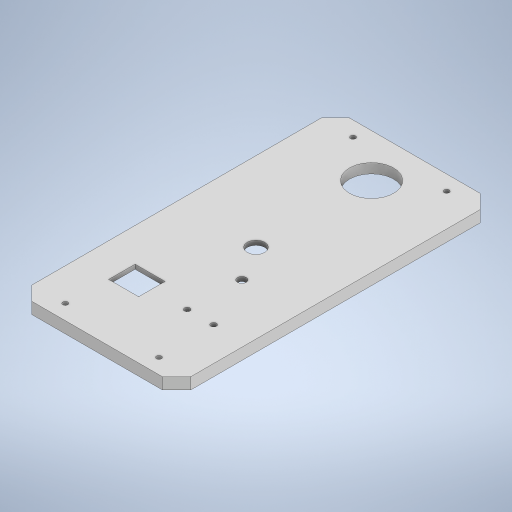
# Autodesk Inventor part: enclosed top
Saved by Autodesk Inventor 2023 (Build 270158000, 158)
## iProperties
Created: 2022-05-30
Part Number: enclosed top
Material: Generic
Document SubType Name: Modeling
Designer: Aakif
Density: 1 g/cm^3
Appearance: Default
Author: Aakif
Autodesk Inventor part; units mm, degrees
ref_plane "YZ Plane" through (0, 0, 0) normal (1, 0, 0) x (0, 1, 0)
ref_plane "XZ Plane" through (0, 0, 0) normal (0, 1, 0) x (-1, 0, 0)
ref_plane "XY Plane" through (0, 0, 0) normal (0, 0, 1) x (1, 0, 0)
sketch "Sketch1" plane through (0, 0, 0) normal (0, 1, 0) x (-1, 0, 0)
  line L0 (37, -90) -> (-37, -90)
  line L1 (-45, -82) -> (-45, 82)
  line L2 (-37, 90) -> (37, 90)
  line L3 (45, 82) -> (45, -82)
  line L4 (45, -90) -> (-45, 90) construction
  line L5 (-45, -90) -> (45, 90) construction
  line L6 (-37, -90) -> (-45, -82)
  line L7 (37, -90) -> (45, -82)
  line L8 (37, 90) -> (45, 82)
  line L9 (-45, 82) -> (-37, 90)
  line L10 (0, 0) -> (0, -65.5)
  circle A0 centre (0, -65.5) radius 12.5
  line L11 (0, 0) -> (0, 0)
  circle A1 centre (0, 0) radius 5
  line L12 (0, 0) -> (17.5, 0)
  line L13 (17.5, 0) -> (17.5, 50)
  line L14 (17.5, 50) -> (0, 50)
  line L15 (0, 50) -> (0, 0)
  line L16 (26, 42.5) -> (9, 42.5)
  line L17 (9, 42.5) -> (9, 57.5)
  line L18 (9, 57.5) -> (26, 57.5)
  line L19 (26, 57.5) -> (26, 42.5)
  line L20 (26, 42.5) -> (9, 57.5) construction
  line L21 (9, 42.5) -> (26, 57.5) construction
  line L22 (9, 50) -> (-11, 50)
  circle A2 centre (-11, 50) radius 1.6
  line L23 (-11, 50) -> (-26, 50)
  circle A3 centre (-26, 50) radius 1.6
  line L24 (41, -80.3431) -> (35.3431, -86)
  line L25 (35.3431, -86) -> (-35.3431, -86)
  line L26 (-35.3431, -86) -> (-41, -80.3431)
  line L27 (-41, -80.3431) -> (-41, 80.3431)
  line L28 (-41, 80.3431) -> (-35.3431, 86)
  line L29 (-35.3431, 86) -> (35.3431, 86)
  line L30 (35.3431, 86) -> (41, 80.3431)
  line L31 (41, 80.3431) -> (41, -80.3431)
  line L32 (45, -90) -> (35.8917, -82.1873)
  circle A4 centre (35.8917, -82.1873) radius 1.45
  circle A5 centre (35.8917, -82.1873) radius 4.45
  line L33 (22.0647, -90) -> (45, -90)
  line L34 (45, -90) -> (45, -77.0647)
  line L35 (45, -77.0647) -> (22.0647, -77.0647)
  line L36 (22.0647, -77.0647) -> (22.0647, -90)
  circle A6 centre (-35.8917, -82.1873) radius 1.45
  circle A7 centre (-35.8917, -82.1873) radius 4.45
  line L37 (-45, -77.0647) -> (-22.0647, -77.0647)
  line L38 (-22.0647, -77.0647) -> (-22.0647, -90)
  circle A8 centre (35.8917, 82.1873) radius 1.45
  circle A9 centre (35.8917, 82.1873) radius 4.45
  line L39 (45, 77.0647) -> (22.0647, 77.0647)
  line L40 (22.0647, 77.0647) -> (22.0647, 90)
  circle A10 centre (-35.8917, 82.1873) radius 4.45
  circle A11 centre (-35.8917, 82.1873) radius 1.45
  line L41 (-45, 77.0647) -> (-22.0647, 77.0647)
  line L42 (-22.0647, 77.0647) -> (-22.0647, 90)
  line L43 (-22.0647, -90) -> (-45, -90)
  line L44 (-45, -90) -> (-45, -77.0647)
  line L45 (-22.0647, 90) -> (-45, 90)
  line L46 (-45, 90) -> (-45, 77.0647)
  line L47 (22.0647, 90) -> (45, 90)
  line L48 (45, 90) -> (45, 77.0647)
  line L49 (0, 0) -> (0, 20)
  line L50 (0, 0) -> (20, 0) construction
  line L51 (0, 20) -> (-12, 20)
  circle A12 centre (-12, 20) radius 2.5
  line L52 (0, 86) -> (12.5, 86)
  line L53 (0, 86) -> (-12.5, 86)
  circle A13 centre (12.5, 86) radius 1.5
  circle A14 centre (-12.5, 86) radius 1.5
  line L54 (0, -65.5) -> (14, -65.5)
  line L55 (0, -65.5) -> (14, -65.5) construction
  line L56 (0, -65.5) -> (-14, -65.5)
  line L57 (0, -65.5) -> (14, -65.5) construction
  circle A15 centre (14, -65.5) radius 0.95
  circle A16 centre (-14, -65.5) radius 0.95
  circle A17 centre (0, -65.5) radius 15.45
  point P0 (22.0647, -86)
  point P1 (-22.0647, -86)
  point P2 (-22.0647, -81.5147)
  point P3 (-26.5147, -77.0647)
  point P4 (-41, -77.0647)
  point P5 (-41, 77.0647)
  point P6 (-26.5147, 77.0647)
  point P7 (-22.0647, 81.5147)
  point P8 (-22.0647, 86)
  point P9 (22.0647, 86)
  point P10 (22.0647, 81.5147)
  point P11 (26.5147, 77.0647)
  point P12 (41, 77.0647)
  point P13 (41, -77.0647)
  point P14 (26.5147, -77.0647)
  point P15 (22.0647, -81.5147)
  point P16 (5, 0)
  point P17 (0, 5)
  point P18 (9, 50)
  point P19 (17.5, 42.5)
  dimension "d0" = 90
  dimension "d1" = 180
  dimension "d2" = 8
  dimension "d3" = 8
  dimension "d4" = 8
  dimension "d5" = 8
  dimension "d6" = 8
  dimension "d7" = 8
  dimension "d8" = 8
  dimension "d9" = 8
  dimension "d10" = 65.5
  dimension "d11" = 25
  dimension "d12" = 0
  dimension "d13" = 10
  dimension "d14" = 17.5
  dimension "d15" = 50
  dimension "d16" = 17
  dimension "d17" = 15
  dimension "d20" = 20
  dimension "d21" = 3.2
  dimension "d22" = 15
  dimension "d23" = 3.2
  dimension "d24" = 4
  dimension "d25" = 12
  dimension "d26" = 2.9
  dimension "d27" = 3
  dimension "d57" = 20
  dimension "d58" = 90
  dimension "d59" = 12
  dimension "d60" = 90
  dimension "d61" = 5
  dimension "d70" = 12.5
  dimension "d71" = 12.5
  dimension "d72" = 3
  dimension "d73" = 3
  dimension "d74" = 14
  dimension "d75" = 0
  dimension "d76" = 14
  dimension "d77" = 180
  dimension "d78" = 1.9
  dimension "d79" = 1.9
  dimension "d80" = 30.9
  constraints: 116 end point, 18 centre point, 14 symmetric about line, 13 point on line, 11 coincident, 10 horizontal, 10 parallel, 8 perpendicular, 6 midpoint, 3 equal length, 2 collinear, 13 other
  measures "d0" distance of L4.end L5.end
  measures "d1" distance of L5.start L4.end
  measures "d2" distance of L0.end L5.start
  measures "d3" distance of L1.start L5.start
  measures "d4" distance of L0.start L4.start
  measures "d5" distance of L3.end L4.start
  measures "d6" distance of L2.end L5.end
  measures "d7" distance of L3.start L5.end
  measures "d8" distance of L1.end L4.end
  measures "d9" distance of L2.start L4.end
  measures "d10" distance of L10.start L10.end
  measures "d11" diameter of A0
  measures "d12" distance of L10.start L11.end
  measures "d13" diameter of A1
  measures "d14" distance of L14.end L13.end
  measures "d15" distance of L13.end L12.end
  measures "d16" distance of L17.end L18.end
  measures "d17" distance of L16.end L17.end
  measures "d20" distance of L22.start L22.end
  measures "d21" diameter of A2
  measures "d22" distance of L23.start L23.end
  measures "d23" diameter of A3
  measures "d24" distance between parallel lines of L7 L24
  measures "d25" distance of L4.start L32.end
  measures "d26" diameter of A4
  measures "d27" radial gap between concentric circles of A4 A5
  measures "d57" distance of L49.start L49.end
  measures "d58" angle of L50 L49
  measures "d59" distance of L49.end L51.end
  measures "d60" angle of L51 L49
  measures "d61" diameter of A12
  measures "d70" distance of L52.start L52.end
  measures "d71" distance of L52.start L53.end
  measures "d72" diameter of A13
  measures "d73" diameter of A14
  measures "d74" distance of L54.start L54.end
  measures "d75" distance between parallel lines of L54 L55
  measures "d76" distance of L54.start L56.end
  measures "d77" angle of L56 L57
  measures "d78" diameter of A15
  measures "d79" diameter of A16
  measures "d80" diameter of A17
extrude "Extrusion1" add sketch "Sketch1" along normal blind 2.5 contours L0 L36 L25 A5 L32 L7 | L0 L38 L25 L36 | L32 A5 L24 L31 L35 L3 L7 | L0 L6 L1 L37 L27 L26 A7 L25 L38 | L36 L35 L31 L24 A5 L25 | L25 L38 L37 L27 L41 L42 L29 A14 A13 L40 L39 L31 L35 L36 | A5 L25 L24 L32 | L32 L24 A5 | L25 A7 L26 L27 L37 L38 | A5 L24 L25 | L35 L31 L39 L3 | A7 L26 L25 | L25 L26 A7 | L39 L31 L30 A9 L29 L40 L2 L8 L3 | L1 L41 L27 L37 | L39 L40 L29 A9 L30 L31 | L1 L9 L2 L42 L29 A10 L28 L27 L41 | L27 L28 A10 L29 L42 L41 | A9 L29 L30 | L30 L29 A9 | L29 A13 A14 L42 L2 L40 | A10 L29 L28 | L28 L29 A10 | A13 L29 | L29 A13 | A14 L29 | L29 A14 | A1 L15 L14 L17 L16 L13 L12 | A4 | A6 | A8 | A11 | A12 | A15 | A16 | A17
sketch "Sketch2" plane through (0, 0, 0) normal (0, -1, 0) x (1, 0, 0)
  line L0 (-26, 57.5) -> (-26, 42.5) projected
  line L1 (-26, 50) -> (-5, 50)
  circle A0 centre (-5, 50) radius 1.45
  circle A1 centre (-5, 50) radius 3.45
  circle A2 centre (0, -65.5) radius 12.5 projected
  line L2 (0, -65.5) -> (-14, -65.5)
  line L3 (0, -65.5) -> (14, -65.5)
  circle A3 centre (-14, -65.5) radius 0.95
  circle A4 centre (14, -65.5) radius 0.95
  circle A5 centre (-14, -65.5) radius 1.45
  circle A6 centre (14, -65.5) radius 1.45
  line L4 (-14, -66.95) -> (-12.3751, -67.2629) construction
  line L5 (-12.3751, -67.2629) -> (-11.6091, -68.4979) construction
  spline S0 degree 2 poles (-14, -66.95) (-12.3751, -67.2629) (-11.6091, -68.4979) knots 1 1 1 2 2 2
  line L6 (-14, -64.05) -> (-12.3751, -63.7371) construction
  line L7 (-12.3751, -63.7371) -> (-11.6091, -62.5021) construction
  spline S1 degree 2 poles (-14, -64.05) (-12.3751, -63.7371) (-11.6091, -62.5021) knots 1 1 1 2 2 2
  line L8 (0, -65.5) -> (0, -61.9317)
  line L9 (14, -66.95) -> (12.3751, -67.2629) construction
  line L10 (12.3751, -67.2629) -> (11.6091, -68.4979) construction
  spline S2 degree 2 poles (14, -66.95) (12.3751, -67.2629) (11.6091, -68.4979) knots 1 1 1 2 2 2
  spline S3 degree 2 poles (14, -64.05) (12.3751, -63.7371) (11.6091, -62.5021) knots 1 1 1 2 2 2
  line L11 (14, -64.05) -> (12.3751, -63.7371) construction
  line L12 (12.3751, -63.7371) -> (11.6091, -62.5021) construction
  circle A7 centre (0, -65.5) radius 12.5
  line L13 (-22.0647, 86) -> (22.0647, 86) projected
  line L14 (0, 60) -> (12.5, 60)
  line L15 (12.5, 60) -> (12.5, 86)
  line L16 (12.5, 86) -> (0, 86)
  line L17 (0, 86) -> (0, 60)
  circle A8 centre (12.5, 86) radius 1.5
  circle A9 centre (-12.5, 86) radius 1.5
  circle A10 centre (0, -65.5) radius 15.45
  point P0 (0, 0)
  point P1 (-12.3047, -67.7011)
  point P2 (-12.3047, -63.2989)
  point P3 (14, -64.05)
  point P4 (12.3047, -63.2989)
  point P5 (12.3047, -67.7011)
  point P6 (-15.45, -65.5)
  point P7 (15.45, -65.5)
  dimension "d30" = 21
  dimension "d31" = 2.9
  dimension "d32" = 2
  dimension "d33" = 14
  dimension "d34" = 14
  dimension "d35" = 1.9
  dimension "d36" = 1.9
  dimension "d37" = 0.5
  dimension "d38" = 0.5
  dimension "d41" = 12.5
  dimension "d42" = 3
  constraints: 16 end point, 10 symmetric about line, 9 centre point, 6 coincident, 4 horizontal, 2 parallel, 1 midpoint, 1 perpendicular, 1 point on line, 1 vertical, 18 other
  measures "d30" distance of L1.start L1.end
  measures "d31" diameter of A0
  measures "d32" radial gap between concentric circles of A0 A1
  measures "d33" distance of L2.start L2.end
  measures "d34" distance of L2.start L3.end
  measures "d35" diameter of A3
  measures "d36" diameter of A4
  measures "d38" radial gap between concentric circles of A4 A6
  measures "d41" distance of L16.end L15.end
  measures "d42" diameter of A8
ref_plane "Work Plane2" through (0, -4, 0) normal (0, -1, 0) x (1, 0, 0)
sketch "Sketch4" plane through (0, -4, 0) normal (0, -1, 0) x (1, 0, 0)
  line L0 (40.0685, -6.5) -> (29.9315, -6.5)
  line L1 (29.9315, -6.5) -> (29.9315, 6.5)
  line L2 (29.9315, 6.5) -> (40.0685, 6.5)
  line L3 (40.0685, 6.5) -> (40.0685, -6.5)
  line L4 (35, 82) -> (35, -82) projected
  line L5 (40.0685, -6.5) -> (29.9315, 6.5) construction
  line L6 (29.9315, -6.5) -> (40.0685, 6.5) construction
  point P0 (0, 0)
  point P1 (35, 0)
  point P2 (35, -6.5)
  point P3 (35, 6.5)
  dimension "d49" = 13
  constraints: 12 end point, 3 midpoint, 2 parallel, 1 horizontal, 1 perpendicular
  measures "d49" distance of L0.end L1.end
ref_plane "Work Plane1" through (0, -4, 0) normal (0, -1, 0) x (1, 0, 0)
sketch "Sketch5" plane through (0, -4, 0) normal (0, -1, 0) x (1, 0, 0)
  circle A0 centre (26.5147, -81.5147) radius 1.45 projected
  circle A1 centre (26.5147, -81.5147) radius 1.45
  circle A2 centre (-26.5147, -81.5147) radius 1.45 projected
  circle A3 centre (-26.5147, -81.5147) radius 1.45
  circle A4 centre (26.5147, 81.5147) radius 1.45 projected
  circle A5 centre (26.5147, 81.5147) radius 1.45
  circle A6 centre (-26.5147, 81.5147) radius 1.45 projected
  circle A7 centre (-26.5147, 81.5147) radius 1.45
  point P0 (0, 0)
  constraints: 4 centre point, 4 coincident
extrude "Extrusion8" add sketch "Sketch1" against normal blind 4 contours L0 L36 L25 A5 L32 L7 | L0 L38 L25 L36 | L32 A5 L24 L31 L35 L3 L7 | L0 L6 L1 L37 L27 L26 A7 L25 L38 | L36 L35 L31 L24 A5 L25 | A5 L25 L24 L32 | L32 L24 A5 | L25 A7 L26 L27 L37 L38 | A5 L24 L25 | L35 L31 L39 L3 | A7 L26 L25 | L25 L26 A7 | L39 L31 L30 A9 L29 L40 L2 L8 L3 | L1 L41 L27 L37 | L39 L40 L29 A9 L30 L31 | L1 L9 L2 L42 L29 A10 L28 L27 L41 | L27 L28 A10 L29 L42 L41 | A9 L29 L30 | L30 L29 A9 | L29 A13 A14 L42 L2 L40 | A10 L29 L28 | L28 L29 A10 | L29 A13 | A14 L29 picked at (11.5718, 86.352) picked at (-13.4282, 86.352)
extrude "Extrusion9" add sketch "Sketch2" along normal blind 3 contours L3 A6 S2 A2 | A2 S3 A6 L3 | A2 S1 A5 A10 A6 S3 | S2 A6 A10 A5 S0 A2 | A6 | A2 L2 A5 S1 | S0 A5 L2 A2 | A5
extrude "Extrusion10" cut sketch "Sketch1" along normal blind 2.5 contours L12 A1 L10 | L15 A1 L12 | L10 A1 L15
extrude "Extrusion11" cut sketch "Sketch1" against normal blind 4 contours L25 L38 L37 L27 L41 L42 L29 A14 A13 L40 L39 L31 L35 L36 | A13 L29 | L29 A14 | L12 A1 L10 | L15 A1 L12 | L10 A1 L15 | A15 | A16 | A17 picked at (11.5145, 85.8803) picked at (-13.4855, 85.8803)
extrude "Extrusion12" add sketch "Sketch1" against normal blind 3 contours A17
extrude "Extrusion13" add sketch "Sketch1" against normal blind 6 contours A13 L29 | L29 A13 | A14 L29 | L29 A14
fillet "Fillet1" radius 3 12 edges at (-41, -2, -77.0647) (-22.0647, -2, 77.0647) (22.0647, -2, -77.0647) (41, -2, -77.0647) (22.0647, -2, -86) (22.0647, -2, 77.0647) (-22.0647, -2, 86) (-41, -2, 77.0647) (41, -2, 77.0647) (22.0647, -2, 86) (-22.0647, -2, -77.0647) (-22.0647, -2, -86)
extrude "Extrusion14" cut sketch "Sketch4" against normal blind 1.5 contours L0 L1 L2 L4
extrude "Extrusion15" cut sketch "Sketch5" against normal blind 6.5
extrude "Extrusion16" cut sketch "Sketch1" along normal blind 2.5 contours A12
equation "\"d3\" = d2"
equation "\"d4\" = d2"
equation "\"d5\" = d4"
equation "\"d6\" = d2"
equation "\"d7\" = d6"
equation "\"d8\" = d2"
equation "\"d9\" = d8"
body "Solid1"
